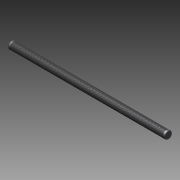
# Autodesk Inventor part: BNT 1605-2.6300 Shaft
Saved by Autodesk Inventor 2011 SP1 (Build 150282100, 282)
## iProperties
Created: 2017-05-16
Part Number: BNT 1605-2.6300 Shaft
Catalog Web Link: www.cadenas.de
Description: BNT Shaft-
Vendor: THK
Document SubType Name: Modeling
Designer: psAdmin
Manufacturer: THK
Mass: 69.5074 g
Surface Area: 180.307 cm^2
Volume: 69.5074 cm^3
Density: 1 g/cm^3
Category: PARTsolutions
Company: THK
Title: BNT 1605-2.6300 Shaft
Author: Cadenas PARTsolutions
PSOL_IDENT_0: {$CADENAS_DATA\23d-libs\thk\fed_screw\ball_screw\ball_screw\standard_lead_rbs\bnt\bnt_shaft.prj},195
PSOL_IDENT_1: {VTYP=3D},{NB=BNT 1605-2.6300 Shaft},{LINA=BNT 1605-2.6300 Shaft},{NN=BNT Shaft},{DATE=22.08.2011 0
PSOL_IDENT_2: 7:52:00},{GEOMDATE=22.08.2011 05:57:00},{VERSION=},{LINEID=10},{LINESUBID=-1},{WBVAR=ST,FS,SS}  {NB=
PSOL_IDENT_3: BNT 1605-2.6300 Shaft},{LINA=BNT 1605-2.6300 Shaft},{KT=DUMMY},{MN=BNT 1605-2.6},{ST=300},{FS=},{SS=
PSOL_IDENT_4: },{OL=346},{EL=1711},{L=36},{R1=9.500},{R2=9.500},{T1=1.800},{T2=1.800},{P3=12.000},{P4=12.000},{B3=
PSOL_IDENT_5: 9.600},{B4=9.600},{G2=3.000},{G3=1.150},{G4=1.150},{F3=9.150},{F4=9.150},{A3=10.000},{A4=10.000},{G1=
PSOL_IDENT_6: 3.000},{S1=14.000},{S2=11.000},{A1=12.000},{A2=12.000},{B1=10.000},{B2=10.000},{J1=13.000},{SD=16},{
PSOL_IDENT_7: J2=13.000},{M1=12.000},{M2=12.000},{P11=1.000},{P2=1.000},{P1=2.000},{FSX='','None','-H1','Type_H1','
PSOL_IDENT_8: -H2','Type_H2','-H3','Type_H3','-J1','Type_J1','-J2','Type_J2','-J3','Type_J3'},{E3=11},{E4=11},{F1=
PSOL_IDENT_9: 15},{E1=39},{N1=6},{H1=8},{F2=15},{E2=36},{N2=6},{H2=8},{STX=1675},{FSX1=0},{SSX1=0},{VERMN=1},{VERK=
PSOL_IDENT_10: 1}
NN: BNT Shaft
NB: BNT 1605-2.6300 Shaft
NBSYN: $MN.$ST.$FS.$SS. Shaft
LINA: BNT 1605-2.6300 Shaft
MN: BNT 1605-2.6
ST: 300
EL: 1711
L: 36
R1: 9.500
R2: 9.500
T1: 1.800
T2: 1.800
P3: 12.000
P4: 12.000
B3: 9.600
B4: 9.600
G2: 3.000
G3: 1.150
G4: 1.150
F3: 9.150
F4: 9.150
A3: 10.000
A4: 10.000
G1: 3.000
S1: 14.000
S2: 11.000
A1: 12.000
A2: 12.000
B1: 10.000
B2: 10.000
J1: 13.000
SD: 16
J2: 13.000
M1: 12.000
M2: 12.000
P11: 1.000
P2: 1.000
P1: 2.000
FSX: '','None','-H1','Type_H1','-H2','Type_H2','-H3','Type_H3','-J1','Type_J1','-J2','Type_J2','-J3','Type_J3'
E3: 11
E4: 11
F1: 15
E1: 39
N1: 6
H1: 8
F2: 15
E2: 36
N2: 6
H2: 8
VERMN: 1
SUPPLIER: THK
ARTICLENO: BNT 1605-2.6300 Shaft
BOMINFO: BNT 1605-2.6300 Shaft
CREATOR: CADENAS GmbH
Autodesk Inventor part; units mm, degrees
ref_plane "YZ Plane" through (0, 0, 0) normal (1, 0, 0) x (0, 1, 0)
ref_plane "XZ Plane" through (0, 0, 0) normal (0, 1, 0) x (-1, 0, 0)
ref_plane "XY Plane" through (0, 0, 0) normal (0, 0, 1) x (1, 0, 0)
sketch "Sketch_1" plane through (0, 0, 0) normal (0, 0, 1) x (1, 0, 0)
  line L0 (341, 0) -> (5, 0)
  line L1 (5, 0) -> (5, 8)
  line L2 (5, 8) -> (341, 8)
  line L3 (341, 8) -> (341, 0)
  line L4 (341, 0) -> (5, 0)
  constraints: 10 end point
revolve "Revolution1" add sketch "Sketch_1" angle 360 about axis through (341, 0, 0) along (1, 0, 0)
thread "Thread1" size "M16x2" class "6g" standard "ISO Metric profile" full length
sketch "Sketch_2" plane through (0, 0, 0) normal (0, 1, 0) x (-1, 0, 0)
  line L0 (-5, 0) -> (0, 0)
  line L1 (0, 0) -> (0, -7.2)
  line L2 (0, -7.2) -> (-0.8, -8)
  line L3 (-0.8, -8) -> (-4.8, -8)
  line L4 (-4.8, -8) -> (-4.8, -6.4)
  line L5 (-4.8, -6.4) -> (-5, -6.4)
  line L6 (-5, -6.4) -> (-5, 0)
  line L7 (-5, 0) -> (0, 0)
  constraints: 16 end point
revolve "Revolution2" add sketch "Sketch_2" angle 360 about axis through (5, 0, 0) along (1, 0, 0)
sketch "Sketch_3" plane through (0, 0, 0) normal (0, 1, 0) x (-1, 0, 0)
  line L0 (-346, 0) -> (-341, 0)
  line L1 (-341, 0) -> (-341, -6.4)
  line L2 (-341, -6.4) -> (-341.2, -6.4)
  line L3 (-341.2, -6.4) -> (-341.2, -8)
  line L4 (-341.2, -8) -> (-345.2, -8)
  line L5 (-345.2, -8) -> (-346, -7.2)
  line L6 (-346, -7.2) -> (-346, 0)
  line L7 (-346, 0) -> (-341, 0)
  constraints: 16 end point
revolve "Revolution3" add sketch "Sketch_3" angle 360 about axis through (346, 0, 0) along (1, 0, 0)
ref_plane "bnt_s_1_XY" through (0, 0, 0) normal (-1, 0, 0) x (0, 0, -1)
ref_plane "bnt_s_1_YZ" through (0, 0, 0) normal (0, 0, -1) x (0, -1, 0)
ref_plane "bnt_s_1_ZX" through (0, 0, 0) normal (0, -1, 0) x (-1, 0, 0)
body "Solid1"
